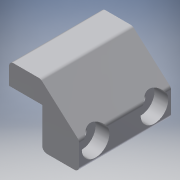
# Autodesk Inventor part: C29_TK_BackWedge
Saved by Autodesk Inventor 2016 (Build 200138000, 138)
## iProperties
Created: 2016-01-30
Part Number: C29_TK_BackWedge
Material: ABS Plastic
Document SubType Name: Modeling
Designer: TheeTimatahee
Density: 1.06 g/cm^3
Appearance: Smooth - White
Mass: 106.755 g
Surface Area: 58.4358 cm^2
Volume: 11.9413 cm^3
Author: TheeTimatahee
Autodesk Inventor part; units mm, degrees
ref_plane "YZ Plane" through (0, 0, 0) normal (1, 0, 0) x (0, 1, 0)
ref_plane "XZ Plane" through (0, 0, 0) normal (0, 1, 0) x (-1, 0, 0)
ref_plane "XY Plane" through (0, 0, 0) normal (0, 0, 1) x (1, 0, 0)
sketch "Sketch1" plane through (0, 0, 0) normal (0, 0, 1) x (1, 0, 0)
  line L0 (-9.2616, -16.795) -> (16.1384, -16.795)
  line L1 (16.1384, -16.795) -> (16.1384, 2.255)
  line L2 (16.1384, 2.255) -> (-10.4396, 25.877)
  line L3 (-10.4396, 25.877) -> (-32.2486, 25.877)
  line L4 (-32.2486, 25.877) -> (-32.2486, 10.891)
  line L5 (-32.2486, 10.891) -> (-9.2616, 10.891)
  line L6 (-9.2616, -16.795) -> (-9.2616, 10.891)
  dimension "d39" = 25.4
  dimension "d40" = 22.987
  dimension "d42" = 27.686
  dimension "d43" = 14.986
  dimension "d45" = 48.37
  dimension "d46" = 19.05
  constraints: 14 end point, 3 perpendicular, 2 vertical, 1 horizontal
  measures "d39" distance of L0.start L0.end
  measures "d40" distance of L4.end L5.end
  measures "d42" distance between parallel lines of L0 L5
  measures "d43" distance of L3.end L4.end
  measures "d45" angle of L6 L2
  measures "d46" distance from line of L0 L1.end
extrude "Extrusion1" add sketch "Sketch1" along normal blind 63.5
sketch "Sketch5" plane through (16.1384, -16.795, 0) normal (1, 0, 0) x (0, 0, -1)
  line L0 (0, 0) -> (-63.5, 0) projected
  line L1 (-63.5, 0) -> (-63.5, 19.05) projected
  line L2 (-63.5, 0) -> (-52.07, 12.7) construction
  line L3 (-52.07, 12.7) -> (-11.43, 12.7) construction
  line L4 (0, 0) -> (0, 19.05) construction
  line L5 (-11.43, 12.7) -> (0, 0) construction
  point P0 (0, 16.795)
  dimension "d47" = 12.7
  dimension "d48" = 11.43
  constraints: 6 end point, 1 equal length, 1 horizontal alignment, 1 perpendicular
  measures "d47" distance from line of L0 L2.end
  measures "d48" distance from line of L1 L2.end
hole "Hole3" at (16.1384, -4.095, 52.07) at (16.1384, -4.095, 11.43) direction (-1, 0, 0) diameter 6.7564 end through all counterbore diameter 19.05 counterbore depth 9.525 clearance for "Hex Head Bolt" size "1/4" standard "Ansi Unified Screw Threads"
fillet "Fillet2" radius 3.175 7 edges at (16.1384, 2.255, 31.75) (16.1384, 2.255, 61.3348) (16.1384, 2.255, 2.1652) (16.1384, -16.795, 31.75) (-9.2616, -16.795, 31.75) (-10.4396, 25.877, 31.75) (-32.2486, 25.877, 31.75)
body "Solid1"
